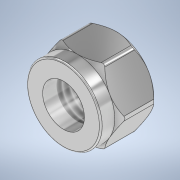
# Autodesk Inventor part: M3_Nylon_Nut
Saved by Autodesk Inventor 2020 (Build 240168000, 168)
## iProperties
Created: 2021-04-28
Part Number: M3_Nylon_Nut
Material: Generic
Document SubType Name: Modeling
Designer: Workshop
Density: 1 g/cm^3
Appearance: Chrome - Polished
Author: Workshop
Autodesk Inventor part; units mm, degrees
ref_plane "YZ Plane" through (0, 0, 0) normal (1, 0, 0) x (0, 1, 0)
ref_plane "XZ Plane" through (0, 0, 0) normal (0, 1, 0) x (-1, 0, 0)
ref_plane "XY Plane" through (0, 0, 0) normal (0, 0, 1) x (1, 0, 0)
sketch "Sketch1" plane through (0, 0, 0) normal (0, 0, 1) x (1, 0, 0)
  line L0 (-3.0888, 0) -> (-1.5444, 2.675)
  line L1 (-1.5444, 2.675) -> (1.5444, 2.675)
  line L2 (1.5444, 2.675) -> (3.0888, 0)
  line L3 (3.0888, 0) -> (1.5444, -2.675)
  line L4 (1.5444, -2.675) -> (-1.5444, -2.675)
  line L5 (-1.5444, -2.675) -> (-3.0888, 0)
  point P0 (0, 0)
  point P1 (0, 0)
  point P2 (0, 2.675)
  dimension "d0" = 5.35
  constraints: 12 end point, 1 coincident, 1 midpoint, 1 vertical alignment, 13 other
  measures "d0" distance between parallel lines of L4 L1
extrude "Extrusion1" add sketch "Sketch1" along normal blind 2.8
sketch "Sketch2" plane through (0, 0, 2.8) normal (0, 0, 1) x (1, 0, 0)
  circle A0 centre (0, 0) radius 2.675
  line L0 (1.5444, 2.675) -> (-1.5444, 2.675) projected
  constraints: 1 centre point, 1 coincident, 1 tangent
extrude "Extrusion2" cut sketch "Sketch2" against normal blind 2.8 draft 45 keep common part
sketch "Sketch3" plane through (0, 0, 0) normal (0, 0, -1) x (-1, 0, 0)
  circle A0 centre (0, 0) radius 2.675
  line L0 (-1.5444, 2.675) -> (1.5444, 2.675) projected
  constraints: 1 centre point, 1 coincident, 1 tangent
extrude "Extrusion3" cut sketch "Sketch3" against normal blind 2.8 draft 45 keep common part
sketch "Sketch4" plane through (0, 0, 2.8) normal (0, 0, 1) x (1, 0, 0)
  circle A0 centre (0, 0) radius 1.5
  dimension "d7" = 3
  constraints: 1 centre point, 1 coincident
  measures "d7" diameter of A0
extrude "Extrusion4" cut sketch "Sketch4" against normal through all
thread "Thread1" size "M3x0.5" class "6H" standard "ANSI Metric M Profile" length 2.8
chamfer "Chamfer1" distance 0.2 angle 45 1 edges at (-1.5, 0, 0)
sketch "Sketch5" plane through (0, 0, 2.8) normal (0, 0, 1) x (1, 0, 0)
  circle A0 centre (0, 0) radius 1.5 projected
  arc A1 (2.3166, 1.3375) -> (0, 2.675) centre (0, 0) ccw projected
  circle A2 centre (0, 0) radius 1.5 projected
  arc A3 (-2.3166, -1.3375) -> (0, -2.675) centre (0, 0) ccw projected
  arc A4 (0, -2.675) -> (2.3166, -1.3375) centre (0, 0) ccw projected
  arc A5 (2.3166, -1.3375) -> (2.3166, 1.3375) centre (0, 0) ccw projected
  arc A6 (2.3166, 1.3375) -> (0, 2.675) centre (0, 0) ccw projected
  arc A7 (0, 2.675) -> (-2.3166, 1.3375) centre (0, 0) ccw projected
  arc A8 (-2.3166, 1.3375) -> (-2.3166, -1.3375) centre (0, 0) ccw projected
  point P0 (0, 2.675)
extrude "Extrusion5" add sketch "Sketch5" along normal blind 1
fillet "Fillet1" radius 0.1 1 edges at (2.3166, 1.3375, 3.8)
fillet "Fillet2" radius 0.3 6 edges at (1.5444, -2.675, 1.4) (3.0888, 0, 1.4) (1.5444, 2.675, 1.4) (-1.5444, 2.675, 1.4) (-3.0888, 0, 1.4) (-1.5444, -2.675, 1.4)
body "Solid1"
